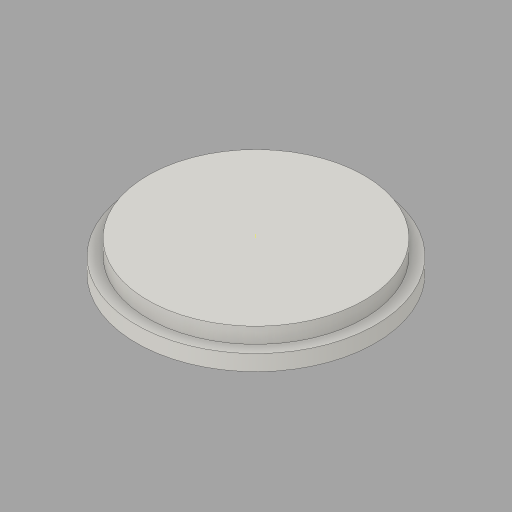
# Autodesk Inventor part: Deckel
Saved by Autodesk Inventor 2023.2 (Build 272271000, 271)
## iProperties
Created: 2023-02-02
Part Number: Deckel
Material: Stahl
Document SubType Name: Modeling
Designer: Raoul Messerli
Density: 7.85 g/cm^3
Appearance: Platte
Author: Raoul Messerli
Autodesk Inventor part; units mm, degrees
ref_plane "YZ Plane" through (0, 0, 0) normal (1, 0, 0) x (0, 1, 0)
ref_plane "XZ Plane" through (0, 0, 0) normal (0, 1, 0) x (-1, 0, 0)
ref_plane "XY Plane" through (0, 0, 0) normal (0, 0, 1) x (1, 0, 0)
sketch "Skizze1" plane through (0, 0, 0) normal (1, 0, 0) x (0, 1, 0)
  line L0 (34.45, 0) -> (34.45, -5)
  line L1 (34.45, -5) -> (38.05, -5)
  line L2 (38.05, -5) -> (38.05, -10)
  line L3 (38.05, -10) -> (0, -10)
  line L4 (0, 0) -> (34.45, 0)
  line L5 (0, 0) -> (0, -10)
  dimension "d1" = 68.9
  dimension "d2" = 76.1
  dimension "d3" = 10
  dimension "d4" = 5
  constraints: 12 end point, 4 perpendicular, 1 vertical
  measures "d1" diameter of L0 L5
  measures "d2" diameter of L2 L5
  measures "d3" distance between parallel lines of L3 L4
  measures "d4" distance of L0.start L0.end
revolve "Umdrehung1" add sketch "Skizze1" angle 360 about axis through (0, 0, 0) along (0, 0, -1)
